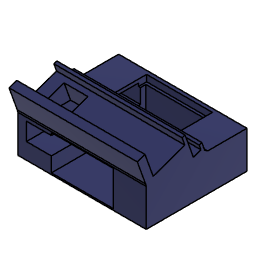
Ups & Downs Enclosure v4 (Autodesk Fusion 360 design; units mm, degrees)
Autodesk Fusion 360 part; units mm, degrees
box "BoxPrimitive1" add length 220 width 220 height 270 placed x (0, -1, 0) y (1, 0, 0) z (0, 0, 1) at (-63.9829, 42.6885, 0) makes body 1
sketch "Sketch3" plane through (0, 0, 0) normal (0, 0, 1) x (1, 0, 0)
  line L0 (0, 0) -> (88, 0)
  line L1 (88, 0) -> (88, -84)
  line L2 (88, -84) -> (0, -84)
  line L3 (0, -84) -> (0, 0)
  dimension "d6" = 88
  dimension "d7" = 84
  constraint horizontal L0
  constraint vertical L1
  constraint horizontal L2
  constraint vertical L3
  constraint coincident L0.start L3.end
  measures "d6" distance of L0.start L0.end
  measures "d7" distance of L0.start L2.end
extrude "Extrude1" add sketch "Sketch3" along normal blind 36 separate body makes body 2
cylinder "CylinderPrimitive1" add diameter 26 height -84 placed x (1, 0, 0) y (0, 0, -1) z (0, 1, 0) at (69.1396, 0, 30.7621) bodies 2
sketch "Sketch6" plane through (0, 0, 0) normal (0, 0, 1) x (1, 0, 0)
  line L0 (0, 0) -> (73, 0)
  line L1 (73, 0) -> (73, -73)
  line L2 (73, -73) -> (0, -73)
  line L3 (0, -73) -> (0, 0)
  dimension "d12" = 73
  dimension "d13" = 73
  constraint horizontal L0
  constraint vertical L1
  constraint horizontal L2
  constraint vertical L3
  constraint coincident L0.start L3.end
  measures "d12" distance of L1.end L2.end
  measures "d13" distance of L0.end L1.end
extrude "Extrude2" add sketch "Sketch6" along normal blind 46 separate body makes body 3
sketch "Sketch7" plane through (0, 0, 0) normal (0, 0, 1) x (1, 0, 0)
  line L0 (0, 0) -> (239, 0)
  line L1 (239, 0) -> (239, -147)
  line L2 (239, -147) -> (0, -147)
  line L3 (0, -147) -> (0, 0)
  dimension "d16" = 239
  dimension "d17" = 147
  constraint horizontal L0
  constraint vertical L1
  constraint horizontal L2
  constraint vertical L3
  constraint coincident L0.start L3.end
  measures "d16" distance of L0.start L0.end
  measures "d17" distance of L0.start L2.end
extrude "Extrude3" add sketch "Sketch7" along normal blind 5 separate body makes body 4
move_body "Move1" bodies 4 to x (1, 0, 0) y (0, 0.34202, -0.939693) z (0, 0.939693, 0.34202) at (0, -6.0327, 16.9096)
move_body "Move2" bodies 2 to x (0, -1, 0) y (1, 0, 0) z (0, 0, 1) at (37.2409, 31.0313, 0)
move_body "Move3" bodies 4 to x (1, 0, 0) y (0, 1, 0) z (0, 0, 1) at (-120.1098, -24.8818, 31.8931)
move_body "Move4" bodies 2 to x (1, 0, 0) y (0, 1, 0) z (0, 0, 1) at (5, 0, 0)
move_body "Move5" bodies 3 to x (1, 0, 0) y (0, -0.34202, 0.939693) z (0, -0.939693, -0.34202) at (-63.5786, -69.2545, 138.9169)
move_body "Move6" bodies 1 to x (1, 0, 0) y (0, 1, 0) z (0, 0, 1) at (-46.6344, 62.1984, 0)
move_body "Move7" bodies 2 3 4 to x (1, 0, 0) y (0, 1, 0) z (0, 0, 1) at (0, 0, 6)
sketch "Sketch9" plane through (0, 0, 0) normal (0, 0, 1) x (1, 0, 0)
  line L0 (-99.0958, 53.0513) -> (99.0958, 53.0513)
  line L1 (99.0958, 53.0513) -> (99.0958, -53.0513)
  line L2 (99.0958, -53.0513) -> (-99.0958, -53.0513)
  line L3 (-99.0958, -53.0513) -> (-99.0958, 53.0513)
  line L4 (-99.0958, 53.0513) -> (99.0958, -53.0513) construction
  line L5 (99.0958, 53.0513) -> (-99.0958, -53.0513) construction
  constraint horizontal L0
  constraint perpendicular L0 L1
  constraint parallel L0 L2
  constraint parallel L1 L3
  constraint coincident L4 origin
  constraint coincident L5 origin
move_body "Move8" bodies 4 3 2 to x (1, 0, 0) y (0, 1, 0) z (0, 0, 1) at (0, 10, 0)
sketch "Sketch10" plane through (0, 0, 0) normal (1, 0, 0) x (0, 1, 0)
  line L0 (53.7068, 0) -> (-87.5847, 0)
  line L1 (-87.5847, 0) -> (-87.5847, 52.2045)
  line L2 (-87.5847, 52.2045) -> (53.7068, 52.2045)
  line L3 (53.7068, 52.2045) -> (53.7068, 0)
  line L4 (-20.6114, 52.2045) -> (-29.3426, 76.802)
  line L5 (-29.3426, 76.802) -> (-88.5742, 55.777)
  line L6 (-88.5742, 55.777) -> (-87.5847, 52.2045)
  line L7 (-7.1136, 59.6082) -> (-23.8558, 53.6653)
  line L8 (-23.8558, 53.6653) -> (-21.0975, 45.8945)
  line L9 (-21.0975, 45.8945) -> (-4.3552, 51.8373)
  line L10 (-4.3552, 51.8373) -> (-7.1136, 59.6082)
  line L11 (-10.7791, 58.307) -> (-13.2277, 65.2054)
  line L12 (-13.2277, 65.2054) -> (-9.5762, 66.5016)
  line L13 (-9.5762, 66.5016) -> (-7.1275, 59.6032)
  line L14 (-7.1275, 59.6032) -> (-10.7791, 58.307)
  line L15 (-29.3426, 76.802) -> (-33.422, 75.354)
  line L16 (-33.422, 75.354) -> (-37.206, 86.014)
  line L17 (-37.206, 86.014) -> (-33.1266, 87.4621)
  line L18 (-33.1266, 87.4621) -> (-29.3426, 76.802)
  line L19 (-77.869, 59.5769) -> (-88.5742, 55.777)
  line L20 (-88.5742, 55.777) -> (-100.066, 88.1514)
  line L21 (-100.066, 88.1514) -> (-89.3608, 91.9514)
  line L22 (-89.3608, 91.9514) -> (-77.869, 59.5769)
  constraint horizontal L0
  constraint vertical L1
  constraint horizontal L2
  constraint vertical L3
  constraint coincident L2 L4.start
  constraint perpendicular L4 L5
  constraint perpendicular L7 L8
  constraint parallel L7 L9
  constraint parallel L8 L10
  constraint perpendicular L4 L7
  constraint perpendicular L11 L12
  constraint parallel L11 L13
  constraint parallel L12 L14
  constraint perpendicular L7 L11
  constraint coincident L7 L11.start
  constraint perpendicular L15 L16
  constraint parallel L15 L17
  constraint parallel L16 L18
  constraint coincident L5 L15.end
  constraint perpendicular L19 L20
  constraint parallel L19 L21
  constraint parallel L20 L22
  constraint parallel L5 L19
extrude "Extrude4" add sketch "Sketch10" along normal blind 90 separate body makes body 5
extrude "Extrude5" add 1 faces at (0, -12.7878, 17.4015) along direction (-1, 0, 0) blind 90 on bodies 5 bodies 5
sketch "Sketch11" plane through (0, 0, 0) normal (0, 1, 0) x (1, 0, 0)
  line L0 (-43.1195, -51.057) -> (43.8805, -51.057)
  line L1 (43.8805, -51.057) -> (43.8805, -2.057)
  line L2 (43.8805, -2.057) -> (-43.1195, -2.057)
  line L3 (-43.1195, -2.057) -> (-43.1195, -51.057)
  dimension "d24" = 49
  dimension "d25" = 87
  constraint horizontal L0
  constraint vertical L1
  constraint horizontal L2
  constraint vertical L3
  measures "d24" distance of L0.start L2.end
  measures "d25" distance of L1.end L2.end
extrude "Extrude6" cut sketch "Sketch11" against normal blind 105 bodies 5
extrude "Extrude7" cut 1 faces at (-14.1195, 0, 34.7236) along direction (0, 1, 0) blind 45 on bodies 5 bodies 5
sketch "Sketch12" plane through (0, 0, 52.2045) normal (0, 0, 1) x (-1, 0, 0)
  line L0 (90, 4.4856) -> (-90, 4.4856)
  line L1 (-90, 4.4856) -> (-90, -53.7068)
  line L2 (-90, -53.7068) -> (90, -53.7068)
  line L3 (90, -53.7068) -> (90, 4.4856)
  line L4 (-46.4713, 3.4134) -> (45.8448, 3.4134)
  line L5 (45.8448, 3.4134) -> (45.8448, -48.7831)
  line L6 (45.8448, -48.7831) -> (-46.4713, -48.7831)
  line L7 (-46.4713, -48.7831) -> (-46.4713, 3.4134)
  constraint horizontal L4
  constraint vertical L5
  constraint horizontal L6
  constraint vertical L7
extrude "Extrude8" cut sketch "Sketch12" against normal blind 9 contours L4 L5 L6 L7 bodies 5
sketch "Sketch14" plane through (0, -87.5847, 0) normal (0, -1, 0) x (1, 0, 0)
  line L0 (-43.1195, 51.057) -> (43.8805, 51.057)
  line L1 (43.8805, 51.057) -> (43.8805, 2.057)
  line L2 (43.8805, 2.057) -> (-43.1195, 2.057)
  line L3 (-43.1195, 2.057) -> (-43.1195, 51.057)
  line L4 (-90, 0) -> (90, 0)
  line L5 (90, 0) -> (90, 52.2045)
  line L6 (90, 52.2045) -> (-90, 52.2045)
  line L7 (-90, 52.2045) -> (-90, 0)
  line L8 (-43.1195, 47.4323) -> (-78.1195, 47.4323)
  line L9 (-78.1195, 47.4323) -> (-78.1195, 22.6741)
  line L10 (-78.1195, 22.6741) -> (-43.1195, 22.6741)
  line L11 (-43.1195, 22.6741) -> (-43.1195, 47.4323)
  dimension "d33" = 35
  constraint horizontal L8
  constraint vertical L9
  constraint horizontal L10
  constraint vertical L11
  constraint coincident L3 L8.start
  measures "d33" distance of L8.start L8.end
extrude "Extrude9" cut sketch "Sketch14" against normal blind 125 contours L3 L8 L9 L10 L11 bodies 5
sketch "Sketch15" plane through (0, -27.4947, 77.4579) normal (0, -0.334514, 0.942391) x (1, 0, 0)
  line L0 (-90, -53.4537) -> (90, -53.4537)
  line L1 (90, -53.4537) -> (90, -6.2896)
  line L2 (90, -6.2896) -> (-90, -6.2896)
  line L3 (-90, -6.2896) -> (-90, -53.4537)
  line L4 (-72.7409, -13.4253) -> (-39.2996, -13.4253)
  line L5 (-39.2996, -13.4253) -> (-39.2996, -43.8154)
  line L6 (-39.2996, -43.8154) -> (-72.7409, -43.8154)
  line L7 (-72.7409, -43.8154) -> (-72.7409, -13.4253)
  constraint horizontal L4
  constraint vertical L5
  constraint horizontal L6
  constraint vertical L7
extrude "Extrude10" cut sketch "Sketch15" against normal blind 30 contours L4 L5 L6 L7 bodies 5
chamfer "Chamfer1" distance 3 angle 45 1 edges at (0, -4.4856, 52.2045) on bodies 5
sketch "Sketch16" plane through (0, -19.5871, 55.1805) normal (0, -0.334514, 0.942391) x (1, 0, 0)
  line L0 (-90, -1.9609) -> (90, -1.9609)
  line L1 (90, -1.9609) -> (90, 9.3464)
  line L2 (90, 9.3464) -> (-90, 9.3464)
  line L3 (-90, 9.3464) -> (-90, -1.9609)
  line L4 (-13.135, 9.3464) -> (13.9936, 9.3464)
  line L5 (13.9936, 9.3464) -> (13.9936, -1.9609)
  line L6 (13.9936, -1.9609) -> (-13.135, -1.9609)
  line L7 (-13.135, -1.9609) -> (-13.135, 9.3464)
  constraint horizontal L4
  constraint vertical L5
  constraint horizontal L6
  constraint vertical L7
  constraint coincident L0 L5.end
  constraint coincident L2 L4.start
extrude "Extrude11" cut sketch "Sketch16" against normal blind 24 contours L0 L2 L4 L5 L6 L7 bodies 5
hidden bodies 2 3 4
named bodies: "Ender 3 S1 Max Build Size", "Printer Silhouette", "PC Silhouette", "Display Silhouette", "Enclosure"
